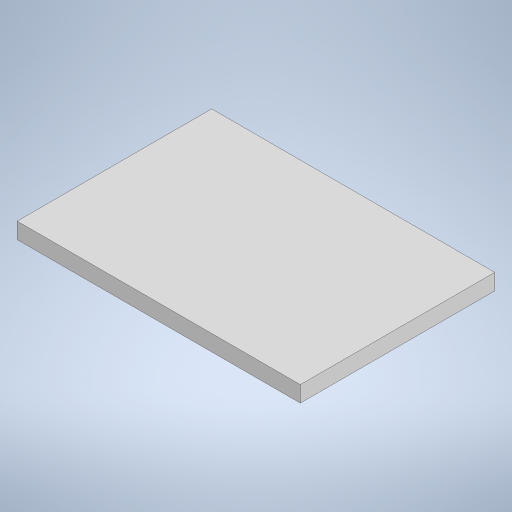
# Autodesk Inventor part: Pieza2
Saved by Autodesk Inventor 2024 (Build 280153000, 153)
## iProperties
Created: 2024-01-31
Part Number: Pieza2
Material: Genérico
Document SubType Name: Modeling
Designer: DANIELA GALEANO
Density: 1 g/cm^3
Appearance: Valor por defecto
Author: DANIELA GALEANO
Autodesk Inventor part; units mm, degrees
ref_plane "YZ Plane" through (0, 0, 0) normal (1, 0, 0) x (0, 1, 0)
ref_plane "XZ Plane" through (0, 0, 0) normal (0, 1, 0) x (-1, 0, 0)
ref_plane "XY Plane" through (0, 0, 0) normal (0, 0, 1) x (1, 0, 0)
sketch "Boceto1" plane through (0, 0, 0) normal (0, 1, 0) x (-1, 0, 0)
  line L0 (8.6276, 15.2812) -> (-256.3724, 15.2812)
  line L1 (-256.3724, 15.2812) -> (-256.3724, -166.7188)
  line L2 (-256.3724, -166.7188) -> (8.6276, -166.7188)
  line L3 (8.6276, -166.7188) -> (8.6276, 15.2812)
  point P0 (0, 0)
  dimension "d0" = 265
  dimension "d1" = 182
  constraints: 8 end point, 2 parallel, 1 horizontal, 1 perpendicular
  measures "d0" distance of L0.start L0.end
  measures "d1" distance of L2.end L0.start
extrude "Extrusión1" add sketch "Boceto1" along normal blind 15
